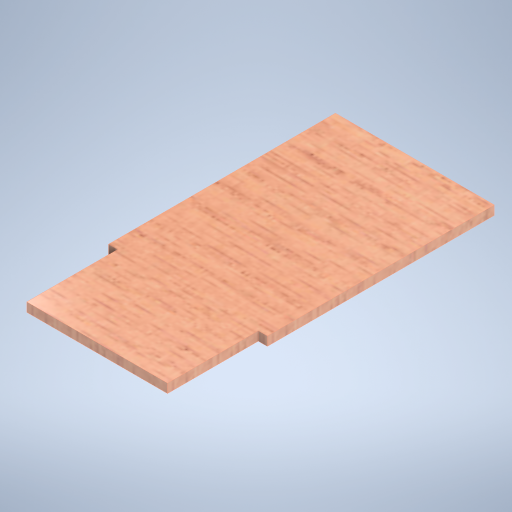
# Autodesk Inventor part: ER_lipo_sikiri
Saved by Autodesk Inventor 2023 (Build 270158000, 158)
## iProperties
Created: 2023-03-05
Part Number: ER_lipo_sikiri
Material: 木材 (オーク)
Document SubType Name: Modeling
Designer: mkhr7
Density: 0.76 g/cm^3
Appearance: ホワイト オーク材 - ナチュラル 標準の光沢
Author: mkhr7
Autodesk Inventor part; units mm, degrees
ref_plane "YZ Plane" through (0, 0, 0) normal (1, 0, 0) x (0, 1, 0)
ref_plane "XZ Plane" through (0, 0, 0) normal (0, 1, 0) x (-1, 0, 0)
ref_plane "XY Plane" through (0, 0, 0) normal (0, 0, 1) x (1, 0, 0)
sketch "スケッチ1" plane through (0, 0, 0) normal (0, 1, 0) x (-1, 0, 0)
  line L0 (0, 0) -> (62, 0)
  line L1 (62, 0) -> (62, -140)
  line L2 (62, -140) -> (0, -140)
  line L3 (0, -140) -> (0, 0)
  line L4 (0, -140) -> (-4, -140)
  line L5 (-4, -140) -> (-4, -40)
  line L6 (-4, -40) -> (0, -40)
  line L7 (0, -40) -> (0, -140)
  line L8 (62, -140) -> (66, -140)
  line L9 (66, -140) -> (66, -40)
  line L10 (66, -40) -> (62, -40)
  line L11 (62, -40) -> (62, -140)
  dimension "d0" = 62
  dimension "d1" = 140
  dimension "d2" = 4
  dimension "d3" = 100
  dimension "d4" = 4
  dimension "d5" = 100
  constraints: 24 end point, 6 parallel, 3 horizontal, 3 perpendicular
  measures "d0" distance of L1.end L2.end
  measures "d1" distance of L0.end L1.end
  measures "d2" distance of L5.end L6.end
  measures "d3" distance of L4.end L5.end
  measures "d4" distance of L10.end L9.end
  measures "d5" distance of L9.end L8.end
extrude "押し出し1" add sketch "スケッチ1" along normal blind 4
